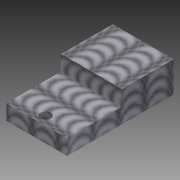
# Autodesk Inventor part: Platine
Saved by Autodesk Inventor 2014 (Build 180170000, 170)
## iProperties
Created: 2013-09-09
Part Number: Platine
Material: Edelstahl
Document SubType Name: Modeling
Designer: vogel
Density: 8.08 g/cm^3
Appearance: Bruchstein - Fluss
Author: vogel
Autodesk Inventor part; units mm, degrees
ref_plane "YZ Plane" through (0, 0, 0) normal (1, 0, 0) x (0, 1, 0)
ref_plane "XZ Plane" through (0, 0, 0) normal (0, 1, 0) x (-1, 0, 0)
ref_plane "XY Plane" through (0, 0, 0) normal (0, 0, 1) x (1, 0, 0)
sketch "Skizze1" plane through (0, 0, 0) normal (0, 0, 1) x (1, 0, 0)
  line L0 (-4, 0) -> (24, 0) projected
  line L1 (0, -7) -> (0, 42) projected
  line L2 (0, 0) -> (20, 0)
  line L3 (20, 0) -> (20, 35)
  line L4 (20, 35) -> (0, 35)
  line L5 (0, 35) -> (0, 0)
  dimension "d0" = 35
  dimension "d1" = 20
  constraints: 8 end point, 2 parallel, 1 horizontal, 1 perpendicular
  measures "d0" distance of L4.end L2.start
  measures "d1" distance of L2.start L2.end
extrude "Extrusion1" add sketch "Skizze1" along normal blind 10
sketch "Skizze2" plane through (0, 0, 10) normal (0, 0, 1) x (1, 0, 0)
  line L0 (0, 0) -> (20, 0) projected
  line L1 (20, 0) -> (20, 35) projected
  point P0 (10, 3)
  dimension "d4" = 10
  dimension "d5" = 3
  measures "d4" distance from line of point (10, 3) L1
  measures "d5" distance from line of point (10, 3) L0
hole "Bohrung1" at (10, 3, 10) direction (0, 0, -1) diameter 3.3 end through all
sketch "Skizze3" plane through (20, 0, 0) normal (1, 0, 0) x (0, 0, -1)
  line L0 (-10, 0) -> (-5, 0)
  line L1 (-5, 0) -> (-5, 18)
  line L2 (-5, 18) -> (-10, 18)
  line L3 (-10, 18) -> (-10, 0)
  dimension "d13" = 5
  dimension "d14" = 18
  constraints: 8 end point, 2 parallel, 1 horizontal, 1 perpendicular
  measures "d13" distance between parallel lines of L3 L1
  measures "d14" distance of L0.end L1.end
extrude "Extrusion2" cut sketch "Skizze3" against normal through all
